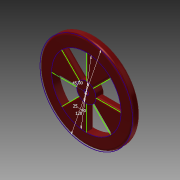
# Autodesk Inventor part: roda_mdf
Saved by Autodesk Inventor 2014 (Build 180170000, 170)
## iProperties
Created: 2015-05-11
Part Number: roda_mdf
Material: Generic
Document SubType Name: Modeling
Designer: Gabriel
Density: 1 g/cm^3
Appearance: Default
Author: Gabriel
Autodesk Inventor part; units mm, degrees
ref_plane "YZ Plane" through (0, 0, 0) normal (1, 0, 0) x (0, 1, 0)
ref_plane "XZ Plane" through (0, 0, 0) normal (0, 1, 0) x (-1, 0, 0)
ref_plane "XY Plane" through (0, 0, 0) normal (0, 0, 1) x (1, 0, 0)
sketch "Sketch1" plane through (0, 0, 0) normal (0, 1, 0) x (-1, 0, 0)
  circle A0 centre (0, 0) radius 3
  circle A1 centre (0, 0) radius 60
  circle A2 centre (0, 0) radius 12.5
  circle A3 centre (0, 0) radius 45
  line L0 (0, -12.5) -> (0, -45)
  line L1 (0, 12.5) -> (0, 45)
  line L2 (-12.5, 0) -> (-45, 0)
  line L3 (12.5, 0) -> (45, 0)
  line L4 (0, 0) -> (5, 0) construction
  line L5 (-8.8388, -8.8388) -> (-31.8198, -31.8198)
  line L6 (8.8388, 8.8388) -> (31.8198, 31.8198)
  line L7 (0, 0) -> (40, 0) construction
  line L8 (-8.8388, 8.8388) -> (-31.8198, 31.8198)
  line L9 (8.8388, -8.8388) -> (31.8198, -31.8198)
  dimension "d4" = 25
  dimension "d5" = 90
  dimension "d0" = 6
  dimension "d1" = 120
  dimension "d7" = 45
  constraints: 20 end point, 4 coincident, 3 collinear, 2 centre point, 2 horizontal, 2 perpendicular, 1 point on line, 1 vertical, 20 other
  measures "d0" diameter of A0
  measures "d1" diameter of A1
  measures "d7" angle of L7 L6
extrude "Extrusion1" add sketch "Sketch1" along normal blind 10 contours A1 | A2 | L3 A3 L9 A2 | A2 L6 A3 L3 | A2 L1 A3 L6 | L9 A3 L0 A2 | A2 L8 A3 L1 | L0 A3 L5 A2 | A2 L2 A3 L8 | L5 A3 L2 A2
extrude "Extrusion2" cut sketch "Sketch1" along normal blind 10 contours L3 A3 L9 A2 | A2 L1 A3 L6 | L0 A3 L5 A2 | A2 L2 A3 L8
fillet "Fillet1" radius 3 2 edges at (60, 0, 0) (60, 10, 0)
fillet "Fillet2" radius 3 16 edges at (28.75, 0, 0) (20.3293, 0, 20.3293) (-20.3293, 0, 20.3293) (-28.75, 0, 0) (-20.3293, 0, -20.3293) (0, 0, -28.75) (20.3293, 0, -20.3293) (41.5746, 10, 17.2208) (20.3293, 10, -20.3293) (0, 10, -28.75) (-20.3293, 10, -20.3293) (-28.75, 10, 0) (-20.3293, 10, 20.3293) (0, 10, 28.75) (28.75, 10, 0) (0, 0, 28.75)
body "Solid1"
